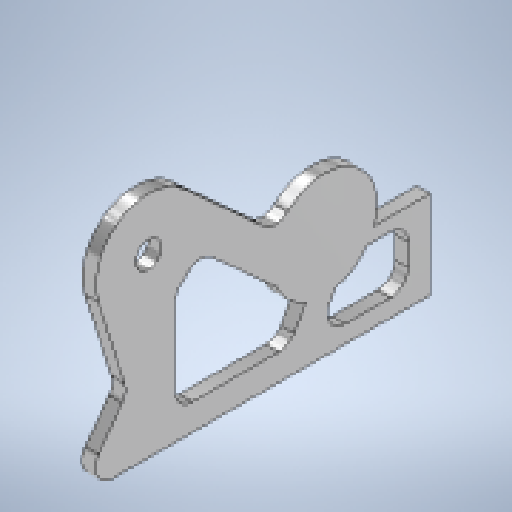
# Autodesk Inventor part: Upright
Saved by Autodesk Inventor 2023.4 (Build 274418000, 418)
## iProperties
Created: 2023-11-13
Part Number: Upright
Material: Aluminum 6061
Document SubType Name: Modeling
Designer: Nathan Cai
Density: 2.7 g/cm^3
Appearance: Aluminum - Flat
Mass: 54.226 g
Surface Area: 113.745 cm^2
Volume: 20.0837 cm^3
Author: Nathan Cai
Autodesk Inventor part; units mm, degrees
ref_plane "YZ Plane" through (0, 0, 0) normal (1, 0, 0) x (0, 1, 0)
ref_plane "XZ Plane" through (0, 0, 0) normal (0, 1, 0) x (-1, 0, 0)
ref_plane "XY Plane" through (0, 0, 0) normal (0, 0, 1) x (1, 0, 0)
sketch "Sketch1" plane through (0, 0, 0) normal (1, 0, 0) x (0, 1, 0)
  circle A0 centre (0, 0) radius 4.7625
  circle A1 centre (0, 0) radius 19.05
  line L0 (-4.2876, 18.5612) -> (-57.15, 6.35)
  line L1 (-57.15, 6.35) -> (-57.15, -101.6)
  circle A2 centre (0, 0) radius 76.2 construction
  line L2 (-57.15, -101.6) -> (-25.4, -101.6)
  line L3 (-25.4, -101.6) -> (-25.4, -63.5)
  line L4 (-25.4, -63.5) -> (-57.15, -45.1691)
  line L5 (-25.4, -63.5) -> (15.0168, -11.7217)
  line L6 (-36.5059, -57.088) -> (-6.0457, -18.0652)
  line L7 (-47.625, -9.525) -> (-47.625, -50.6684)
  line L8 (-30.1625, -71.7489) -> (-57.15, -56.1677)
  line L9 (-30.1625, -71.7489) -> (-30.1625, -93.6625)
  line L10 (-30.1625, -93.6625) -> (-50.8, -93.6625)
  line L11 (-50.8, -93.6625) -> (-50.8, -59.8338)
  line L12 (-47.625, -9.525) -> (-16.4978, -9.525)
  line L13 (-57.15, 6.35) -> (-25.4, 6.35)
  line L14 (-25.4, 6.35) -> (-25.4, 31.75) construction
  line L15 (-25.4, 31.75) -> (-57.15, 31.75) construction
  line L16 (-57.15, 31.75) -> (-57.15, 6.35)
  line L17 (-25.4, 6.35) -> (-57.15, 31.75)
  line L18 (-25.4, -101.6) -> (-16.4555, -90.7388)
  line L19 (-16.4555, -90.7388) -> (17.6378, -7.198)
  point P0 (-32.5137, 12.041)
  point P1 (-47.625, -9.525)
  dimension "d0" = 9.525
  dimension "d2" = 38.1
  dimension "d3" = 107.95
  dimension "d4" = 152.4
  dimension "d5" = 31.75
  dimension "d6" = 38.1
  dimension "d7" = 60
  dimension "d9" = 12.7
  dimension "d10" = 9.525
  dimension "d11" = 9.525
  dimension "d12" = 7.9375
  dimension "d13" = 6.35
  dimension "d14" = 4.7625
  dimension "d19" = 31.75
  dimension "d20" = 25.4
  dimension "d32" = 57.15
  dimension "d33" = 6.35
  dimension "d34" = 9.525
  constraints: 40 end point, 5 parallel, 5 point on circle, 5 point on line, 4 perpendicular, 3 centre point, 3 coincident, 3 tangent, 2 horizontal, 1 vertical, 4 other
  measures "d0" diameter of A0
  measures "d2" diameter of A1
  measures "d3" distance of L0.end L1.end
  measures "d4" diameter of A2
  measures "d5" distance of L1.end L2.end
  measures "d6" distance of L2.end L3.end
  measures "d7" angle of L1 L4
  measures "d9" distance between parallel lines of L5 L6
  measures "d10" distance between parallel lines of L1 L7
  measures "d11" distance between parallel lines of L4 L8
  measures "d12" distance between parallel lines of L2 L10
  measures "d13" distance between parallel lines of L1 L11
  measures "d14" distance between parallel lines of L3 L9
  measures "d19" distance of L15.end L14.end
  measures "d20" distance of L14.end L13.end
  measures "d32" distance from line of L1 point (0, 0)
  measures "d33" distance from line of point (0, 0) L13
  measures "d34" distance from line of point (0, 0) L12
extrude "Extrusion1" add sketch "Sketch1" along normal blind 4.7625 contours A1 | A1 L12 L7 L4 L1 L13 L17 L0 | L17 L13 L0 | L0 L16 L17 | L5 L4 L6 A1 | L3 L2 L1 L4
fillet "Fillet1" radius 6.35 10 edges at (2.3813, -6.0457, -18.0652) (2.3813, -16.4978, -9.525) (2.3813, -36.5059, -57.088) (2.3813, -47.625, -50.6684) (2.3813, -50.8, -59.8338) (2.3813, -30.1625, -71.7489) (2.3813, -30.1625, -93.6625) (2.3813, -50.8, -93.6625) (2.3813, -25.4, -63.5) (2.3813, -47.625, -9.525)
fillet "Fillet2" radius 6.35 2 edges at (2.3813, -57.15, 31.75) (2.3813, -32.5137, 12.041)
sketch "Sketch2" plane through (0, 0, 0) normal (-1, 0, 0) x (0, 0, 1)
  circle A0 centre (0, 0) radius 11.1125
  dimension "d24" = 22.225
  constraints: 1 centre point, 1 coincident
  measures "d24" diameter of A0
equation "\"d9\" = d8"
equation "\"d19\" = d5"
equation "\"d8\" = 12.7"
body "Solid1"
